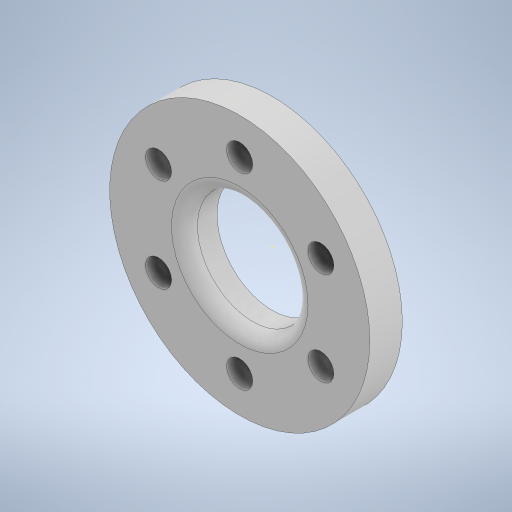
# Autodesk Inventor part: RODADURA NUEVA 222
Saved by Autodesk Inventor 2024.2 (Build 282272000, 272)
## iProperties
Created: 2024-03-30
Part Number: RODADURA NUEVA 222
Material: Generic
Document SubType Name: Modeling
Designer: luisf
Density: 1 g/cm^3
Appearance: Default
Author: luisf
Autodesk Inventor part; units mm, degrees
ref_plane "YZ Plane" through (0, 0, 0) normal (1, 0, 0) x (0, 1, 0)
ref_plane "XZ Plane" through (0, 0, 0) normal (0, 1, 0) x (-1, 0, 0)
ref_plane "XY Plane" through (0, 0, 0) normal (0, 0, 1) x (1, 0, 0)
sketch "Sketch1" plane through (0, 0, 0) normal (0, 0, 1) x (1, 0, 0)
  point P0 (0, 0)
sketch "Sketch2" plane through (0, 0, 0) normal (0, 0, 1) x (1, 0, 0)
  circle A0 centre (0, 0) radius 40
  circle A1 centre (0, 0) radius 17
  circle A2 centre (0, 28.8143) radius 4
  circle A3 centre (-24.9539, 14.4071) radius 4
  circle A4 centre (-24.9539, -14.4071) radius 4
  circle A5 centre (0, -28.8143) radius 4
  circle A6 centre (24.9539, -14.4071) radius 4
  circle A7 centre (24.9539, 14.4071) radius 4
  dimension "d0" = 80
  dimension "d1" = 34
  dimension "d2" = 8
  dimension "d5" = 360
  constraints: 8 centre point, 2 coincident, 1 vertical alignment, 13 other
  measures "d0" diameter of A0
  measures "d1" diameter of A1
  measures "d2" diameter of A2
extrude "Extrusion1" add sketch "Sketch2" along normal blind 10
fillet "Fillet1" radius 4 1 edges at (-17, 0, 10)
body "Solid1"
